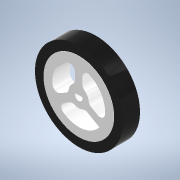
# Autodesk Inventor part: front wheel v2
Saved by Autodesk Inventor 2022.6 (Build 266554000, 554)
## iProperties
Created: 2024-08-28
Part Number: front wheel v2
Material: Generic
Document SubType Name: Modeling
Designer: david
Density: 1 g/cm^3
Appearance: Smooth - White
Author: david
Autodesk Inventor part; units mm, degrees
ref_plane "YZ Plane" through (0, 0, 0) normal (1, 0, 0) x (0, 1, 0)
ref_plane "XZ Plane" through (0, 0, 0) normal (0, 1, 0) x (-1, 0, 0)
ref_plane "XY Plane" through (0, 0, 0) normal (0, 0, 1) x (1, 0, 0)
sketch "Sketch1" plane through (0, 0, 0) normal (0, 0, 1) x (1, 0, 0)
  circle A0 centre (0, 0) radius 17.5
  dimension "d0" = 35
  constraints: 1 centre point, 1 coincident
  measures "d0" diameter of A0
extrude "Extrusion1" add sketch "Sketch1" along normal mid plane 7
sketch "Sketch2" plane through (0, 0, 3.5) normal (0, 0, 1) x (1, 0, 0)
  circle A0 centre (0, 0) radius 10.5
  circle A1 centre (0, 0) radius 4
  line L0 (1.5, 0) -> (-1.5, 0)
  line L1 (-1.5, 0) -> (-1.5, 10.5)
  line L2 (-1.5, 10.5) -> (1.5, 10.5)
  line L3 (1.5, 10.5) -> (1.5, 0)
  line L4 (0.75, -1.299) -> (-8.3433, -6.549)
  line L5 (-9.8433, -3.951) -> (-0.75, 1.299)
  line L6 (0.75, 1.299) -> (9.8433, -3.951)
  line L7 (8.3433, -6.549) -> (-0.75, -1.299)
  point P0 (0, 10.5)
  point P1 (8.25, -6.4952)
  point P2 (2.4613, -3.1531)
  point P3 (-2.4613, -3.1531)
  point P4 (-8.25, -6.4952)
  point P5 (3.9613, -0.555)
  point P6 (9.75, -3.8971)
  point P7 (1.5, 10.3923)
  point P8 (1.5, 3.7081)
  point P9 (-9.75, -3.8971)
  point P10 (-3.9613, -0.555)
  point P11 (-1.5, 3.7081)
  point P12 (-1.5, 10.3923)
  dimension "d3" = 21
  dimension "d4" = 8
  dimension "d5" = 3
  dimension "d8" = 360
  constraints: 16 end point, 2 centre point, 2 coincident, 2 parallel, 1 horizontal, 1 horizontal alignment, 1 midpoint, 1 perpendicular, 1 tangent, 1 vertical alignment, 19 other
  measures "d3" diameter of A0
  measures "d4" diameter of A1
  measures "d5" distance of L1.end L2.end
extrude "Extrusion2" cut sketch "Sketch2" against normal through all contours A0 L6 A1 L3 | A0 L4 A1 L7 | L1 A1 L5 A0
fillet "Fillet1" radius 2 11 edges at (1.5, 3.7081, 0) (3.9613, -0.555, 0) (9.75, -3.8971, 0) (-8.25, -6.4952, 0) (-9.75, -3.8971, 0) (-3.9613, -0.555, 0) (-1.5, 3.7081, 0) (1.5, 10.3923, 0) (-1.5, 10.3923, 0) (-2.4613, -3.1531, 0) (2.4613, -3.1531, 0)
sketch "Sketch4" plane through (0, 0, -3.5) normal (0, 0, -1) x (-1, 0, 0)
  circle A0 centre (0, 0) radius 4
  arc A1 (3.9803, 0.3963) -> (2.3333, 3.2489) centre (0, 0) ccw projected
  constraints: 1 centre point, 1 coincident, 1 concentric
extrude "Extrusion4" add sketch "Sketch4" along normal blind 2
sketch "Sketch3" plane through (0, 0, 3.5) normal (0, 0, 1) x (1, 0, 0)
  circle A0 centre (0, 0) radius 1.5
  line L0 (1.4142, 0.5) -> (-1.4142, 0.5)
  dimension "d17" = 3
  dimension "d19" = 2
  constraints: 2 end point, 2 point on circle, 1 centre point, 1 coincident, 1 horizontal
  measures "d17" diameter of A0
extrude "Extrusion3" cut sketch "Sketch3" against normal through all contours A0 L0 picked at (0.0393, -0.1651)
sketch "Sketch5" plane through (0, 0, 3.5) normal (0, 0, 1) x (1, 0, 0)
  circle A0 centre (0, 0) radius 14
  circle A1 centre (0, 0) radius 17.5 projected
  dimension "d22" = 28
  constraints: 1 centre point, 1 coincident
  measures "d22" diameter of A0
extrude "Extrusion5" cut sketch "Sketch5" against normal blind 0.1
mirror "Mirror1" about plane through (0, 0, 0) normal (0, 0, 1) of "Extrusion5"
body "Solid1"
